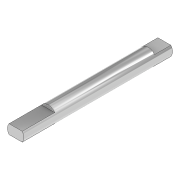
# Autodesk Inventor part: 5x45.75mm Rod
Saved by Autodesk Inventor 2020 (Build 240168000, 168)
## iProperties
Created: 2021-06-26
Part Number: 5x45.75mm Rod
Material: Generic
Document SubType Name: Modeling
Designer: Coy
Density: 1 g/cm^3
Appearance: Chrome - Polished
Author: Coy
Autodesk Inventor part; units mm, degrees
ref_plane "YZ Plane" through (0, 0, 0) normal (1, 0, 0) x (0, 1, 0)
ref_plane "XZ Plane" through (0, 0, 0) normal (0, 1, 0) x (-1, 0, 0)
ref_plane "XY Plane" through (0, 0, 0) normal (0, 0, 1) x (1, 0, 0)
sketch "Sketch1" plane through (0, 0, 0) normal (0, 0, 1) x (1, 0, 0)
  circle A0 centre (0, 0) radius 2.5
  dimension "d0" = 5
  constraints: 1 centre point, 1 coincident
  measures "d0" diameter of A0
extrude "Extrusion1" add sketch "Sketch1" against normal blind 45.75
sketch "Sketch2" plane through (0, 0, -45.75) normal (0, 0, -1) x (-1, 0, 0)
  line L0 (-10.2354, 1.5) -> (9.3002, 1.5)
  line L1 (-10.2354, -1.5) -> (9.3002, -1.5)
  circle A0 centre (0, 0) radius 2.5 projected
  point P0 (2, 1.5)
  point P1 (-2, 1.5)
  point P2 (2, -1.5)
  point P3 (-2, -1.5)
  dimension "d3" = 1.5
  dimension "d4" = 3
  constraints: 4 end point, 2 horizontal
  measures "d3" distance from line of L1 point (0, 0)
  measures "d4" distance between parallel lines of L0 L1
extrude "Extrusion2" cut sketch "Sketch2" against normal blind 5 contours A0 L0 | L1 A0
sketch "Sketch3" plane through (0, 0, 0) normal (0, 0, 1) x (1, 0, 0)
  line L0 (-6.8963, 1.45) -> (8.8768, 1.45)
  line L1 (8.8775, -1.45) -> (-6.8971, -1.45)
  circle A0 centre (0, 0) radius 2.5 projected
  point P0 (-2.0365, -1.45)
  point P1 (2.0365, -1.45)
  point P2 (2.0365, 1.45)
  point P3 (-2.0365, 1.45)
  dimension "d7" = 2.9
  dimension "d8" = 1.45
  constraints: 4 end point, 2 horizontal
  measures "d7" distance between parallel lines of L1 L0
  measures "d8" distance from line of point (0, 0) L0
extrude "Extrusion3" cut sketch "Sketch3" against normal blind 10 contours A0 L0 | L1 A0
equation "\"d8\" = 0.5 * d7"
body "Solid1"
